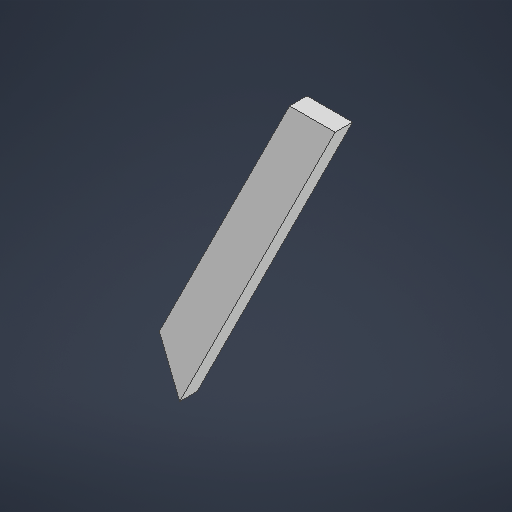
# Autodesk Inventor part: S_2x4x29.814
Saved by Autodesk Inventor 2026 (Build 300175000, 175)
## iProperties
Created: 2025-09-04
Part Number: S_2x4x29.814
Material: Generic
Document SubType Name: Modeling
Designer: trott
Density: 1 g/cm^3
Appearance: Default
Author: trott
Autodesk Inventor part; units mm, degrees
ref_plane "YZ Plane" through (0, 0, 0) normal (1, 0, 0) x (0, 1, 0)
ref_plane "XZ Plane" through (0, 0, 0) normal (0, 1, 0) x (-1, 0, 0)
ref_plane "XY Plane" through (0, 0, 0) normal (0, 0, 1) x (1, 0, 0)
sketch "Sketch1" plane through (0, 0, 0) normal (0, 0, 1) x (1, 0, 0)
  line L0 (0, 0) -> (0, 1524)
  line L1 (0, 1524) -> (0, 1828.8)
  line L2 (0, 0) -> (609.6, 0)
  line L3 (609.6, 0) -> (1219.2, 0)
  line L4 (609.6, 0) -> (609.6, 1524)
  line L5 (609.6, 1524) -> (0, 1524)
  line L6 (0, 1828.8) -> (609.6, 1524)
  line L7 (609.6, 1524) -> (1219.2, 0)
  line L8 (609.6, 1524) -> (1219.2, 1524)
  line L9 (1219.2, 1524) -> (1219.2, 2133.6)
  line L10 (1219.2, 2133.6) -> (1130.3, 2111.375)
  line L11 (1219.2, 2133.6) -> (1130.3, 2133.6)
  line L12 (1130.3, 2133.6) -> (1130.3, 1524)
  line L13 (0, 1828.8) -> (21.5614, 1742.5543)
  line L14 (1130.3, 2111.375) -> (1151.8614, 2025.1293)
  line L15 (21.5614, 1742.5543) -> (1151.8614, 2025.1293)
  line L16 (1130.3, 2111.375) -> (0, 1828.8)
  line L17 (1219.2, 1524) -> (1219.2, 914.4)
  line L18 (1219.2, 914.4) -> (914.4, 914.4)
  line L19 (914.4, 914.4) -> (1219.2, 1524)
  line L20 (914.4, 914.4) -> (880.5333, 846.6667)
  line L21 (880.5333, 846.6667) -> (801.0188, 886.424)
  line L22 (1219.2, 1524) -> (1139.6854, 1563.7573)
  line L23 (1139.6854, 1563.7573) -> (801.0188, 886.424)
  point P0 (1119.8068, 1524)
  point P1 (836.3586, 957.1036)
  dimension "d40" = 1524
  dimension "d41" = 304.8
  dimension "d42" = 609.6
  dimension "d43" = 609.6
  dimension "d44" = 1524
  dimension "d45" = 609.6
  dimension "d46" = 609.6
  dimension "d47" = 88.9
  dimension "d48" = 88.9
  dimension "d49" = 90
  dimension "d50" = 88.9
  dimension "d51" = 90
  dimension "d52" = 609.6
  dimension "d53" = 304.8
  dimension "d54" = 88.9
  dimension "d55" = 88.9
  dimension "d56" = 90
  dimension "d57" = 90
  constraints: 48 end point, 8 point on line, 3 perpendicular, 3 vertical, 1 horizontal, 1 parallel
  measures "d40" distance of L0.start L0.end
  measures "d41" distance of L0.end L1.end
  measures "d42" distance of L0.start L2.end
  measures "d43" distance of L2.end L3.end
  measures "d44" distance of L2.end L4.end
  measures "d45" distance of L4.end L8.end
  measures "d46" distance of L8.end L9.end
  measures "d47" distance of L9.end L11.end
  measures "d48" distance of L1.end L13.end
  measures "d49" angle of L10 L13
  measures "d50" distance of L10.end L14.end
  measures "d51" angle of L10 L14
  measures "d52" distance of L8.end L17.end
  measures "d53" distance of L17.end L18.end
  measures "d54" distance of L20.end L21.end
  measures "d55" distance of L8.end L22.end
  measures "d56" angle of L19 L22
  measures "d57" angle of L20 L21
extrude "Extrusion2" add sketch "Sketch1" along normal blind 38.1 contours L23 L8 L19 L20 L7
body "Solid2"
